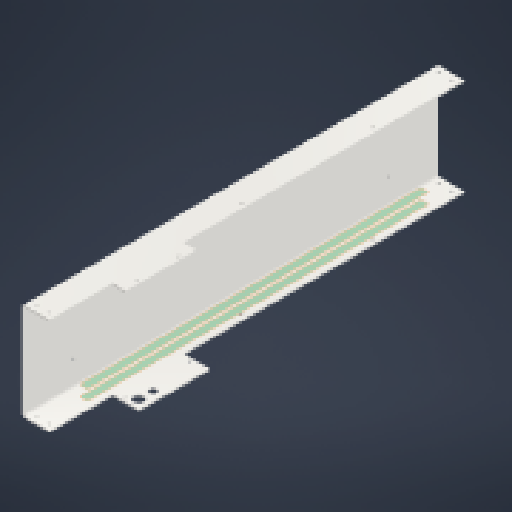
# Autodesk Inventor part: U-Blech-Bild
Saved by Autodesk Inventor 2026.1 (Build 301233020, 233B)
## iProperties
Created: 2025-04-28
Part Number: U-Blech-Bild
Material: Stahl, unlegiert
Document SubType Name: Sheet Metal
Designer: iopeter
Density: 7.85 g/cm^3
Sheet Metal Rule: Standard_mm
Appearance: Stahl
Author: iopeter
Autodesk Inventor part; units mm, degrees
ref_plane "YZ Plane" through (0, 0, 0) normal (1, 0, 0) x (0, 1, 0)
ref_plane "XZ Plane" through (0, 0, 0) normal (0, 1, 0) x (-1, 0, 0)
ref_plane "XY Plane" through (0, 0, 0) normal (0, 0, 1) x (1, 0, 0)
sketch "Skizze1" plane through (0, 0, 0) normal (0, 0, 1) x (1, 0, 0)
  line L0 (26.7, -375) -> (-26.6, -375)
  line L1 (-26.6, -375) -> (-26.6, 415)
  line L2 (-26.6, 415) -> (26.7, 415)
  line L3 (26.7, 415) -> (26.7, -375)
  line L4 (26.7, -120) -> (51.7, -120)
  line L5 (51.7, -120) -> (51.7, -255)
  line L6 (51.7, -255) -> (26.7, -255)
  line L7 (26.7, -255) -> (26.7, -120)
  line L8 (44.7, -147) -> (44.7, -148) construction
  line L9 (42.2, -147) -> (42.2, -148)
  line L10 (47.2, -148) -> (47.2, -147)
  arc A0 (47.2, -147) -> (42.2, -147) centre (44.7, -147) ccw
  arc A1 (42.2, -148) -> (47.2, -148) centre (44.7, -148) ccw
  line L11 (44.7, -227) -> (44.7, -228) construction
  line L12 (42.2, -227) -> (42.2, -228)
  line L13 (47.2, -228) -> (47.2, -227)
  arc A2 (47.2, -227) -> (42.2, -227) centre (44.7, -227) ccw
  arc A3 (42.2, -228) -> (47.2, -228) centre (44.7, -228) ccw
  line L14 (57.888, -187.5) -> (31.6499, -187.5) construction
  line L15 (16.7, 278.8638) -> (16.7, -278.8638) construction
  circle A4 centre (16.7, 250) radius 3
  circle A5 centre (16.7, 0) radius 3
  circle A6 centre (16.7, -250) radius 3
  point P0 (0, 0)
  point P1 (44.7, -147.5)
  point P2 (44.7, -227.5)
  dimension "d17" = 135
  dimension "d19" = 1
  dimension "d20" = 5
  dimension "d21" = 1
  dimension "d22" = 5
  dimension "d23" = 7
  dimension "d24" = 80
  dimension "d26" = 250
  dimension "d28" = 6
  dimension "d29" = 6
  dimension "d30" = 6
  dimension "d52" = 120
  dimension "d63" = 790
  dimension "d65" = 25
  dimension "d67" = 53.3
  dimension "d68" = 375
  dimension "d69" = 26.6
  dimension "d70" = 10
  dimension "d71" = 250
  measures "d17" distance between parallel lines of L6 L4
  measures "d19" distance of L8.start L8.end
  measures "d20" diameter of A1
  measures "d21" distance of L11.start L11.end
  measures "d22" diameter of A3
  measures "d23" distance from line of L5 point (44.7, -147.5)
  measures "d24" distance of point (44.7, -227.5) point (44.7, -147.5)
  measures "d26" distance of point (16.7, 250) point (16.7, 0)
  measures "d28" diameter of A4
  measures "d29" diameter of A5
  measures "d30" diameter of A6
  measures "d52" distance between parallel lines of L0 L6
  measures "d63" distance between parallel lines of L2 L0
  measures "d65" distance between parallel lines of L3 L5
  measures "d67" distance between parallel lines of L1 L3
  measures "d68" distance from line of point (0, 0) L0
  measures "d69" distance from line of L1 point (0, 0)
  measures "d70" distance between parallel lines of L3 L15
  measures "d71" vertical distance of point (0, 0) A6.centre
extrude "Grobblech1" add sketch "Skizze1" along normal blind 3 contours L0 L1 L2 L3 | L3 L4 L5 L6 | A6
ref_plane "Arbeitsebene1" through (13.4, 0, -160) normal (0, 0, -1) x (-1, 0, 0)
ref_plane "Work Plane2" through (13.4, 0, -180) normal (0, 0, -1) x (-1, 0, 0)
sketch "Skizze2" plane through (13.4, 0, -180) normal (0, 0, -1) x (-1, 0, 0)
  circle A0 centre (-3.3, 250) radius 3
  circle A1 centre (-3.3, 0) radius 3
  circle A2 centre (-3.3, -250) radius 3
  circle A3 centre (-3.3, 250) radius 3
  circle A4 centre (-3.3, 0) radius 3
  arc A5 (-33.8, -228) -> (-28.8, -228) centre (-31.3, -228) ccw construction
  line L0 (-28.8, -228) -> (-28.8, -227) construction
  arc A6 (-28.8, -227) -> (-33.8, -227) centre (-31.3, -227) ccw construction
  line L1 (-33.8, -227) -> (-33.8, -228) construction
  line L2 (-33.8, -147) -> (-33.8, -148) construction
  arc A7 (-33.8, -148) -> (-28.8, -148) centre (-31.3, -148) ccw construction
  line L3 (-28.8, -148) -> (-28.8, -147) construction
  arc A8 (-28.8, -147) -> (-33.8, -147) centre (-31.3, -147) ccw construction
  line L4 (-38.3, -120) -> (-38.3, -255)
  line L5 (-13.3, -120) -> (-38.3, -120)
  line L6 (-13.3, 415) -> (-13.3, -120)
  line L7 (40, 415) -> (-13.3, 415)
  line L8 (40, -375) -> (40, 415)
  line L9 (-13.3, -375) -> (40, -375)
  line L10 (-13.3, -255) -> (-13.3, -375)
  line L11 (-38.3, -255) -> (-13.3, -255)
  line L12 (-38.3, -255) -> (-63.3, -255)
  line L13 (-63.3, -255) -> (-63.3, -120)
  line L14 (-63.3, -120) -> (-38.3, -120)
  line L15 (-38.3, -120) -> (-38.3, -255)
  circle A9 centre (-45.3, -237) radius 10.375
  line L16 (-46.078, -226.6542) -> (-44.522, -226.6542)
  line L17 (-31.3, -228) -> (-31.3, -262.846) construction
  circle A10 centre (-31.3, -249) radius 2.5
  line L18 (-38.3, -255) -> (-38.3, -120)
  line L19 (-38.3, -187.5) -> (-17.972, -187.5) construction
  line L20 (-31.3, -147) -> (-31.3, -112.154) construction
  circle A11 centre (-31.3, -126) radius 2.5
  circle A12 centre (-45.3, -210) radius 8.05
  circle A13 centre (-45.3, -210) radius 11 construction
  line L21 (-55.8532, -247.1825) -> (-59.3949, -232.9519) construction
  line L22 (-59.3949, -232.9519) -> (-48.8417, -222.7694) construction
  line L23 (-48.8417, -222.7694) -> (-34.7468, -226.8175) construction
  line L24 (-34.7468, -226.8175) -> (-31.2051, -241.0481) construction
  line L25 (-31.2051, -241.0481) -> (-41.7583, -251.2306) construction
  line L26 (-41.7583, -251.2306) -> (-55.8532, -247.1825) construction
  circle A14 centre (-45.3, -237) radius 14.6647 construction
  line L27 (-37.25, -203.225) -> (-53.35, -203.225)
  line L28 (-53.35, -203.225) -> (-53.35, -216.775)
  line L29 (-53.35, -216.775) -> (-37.25, -216.775)
  line L30 (-37.25, -216.775) -> (-37.25, -203.225)
  line L31 (-37.25, -203.225) -> (-53.35, -216.775) construction
  line L32 (-53.35, -203.225) -> (-37.25, -216.775) construction
  line L33 (-50.7634, -228.18) -> (-39.8366, -228.18)
  point P0 (13.4, 0)
  point P1 (-38.3, -244.6577)
  point P2 (-38.3, -229.3423)
  point P3 (-53.35, -210)
  point P4 (-49.6476, -203.225)
  point P5 (-40.9524, -203.225)
  point P6 (-40.9524, -216.775)
  point P7 (-49.6476, -216.775)
  dimension "d53" = 25
  dimension "d55" = 20.75
  dimension "d57" = 18
  dimension "d58" = 18
  dimension "d59" = 5
  dimension "d60" = 6
  dimension "d61" = 16.1
  dimension "d62" = 27
  dimension "d75" = 22
  dimension "d76" = 25.4
  dimension "d77" = 13.55
  dimension "d78" = 8.82
  measures "d53" distance of L13.end L14.end
  measures "d55" diameter of A9
  measures "d57" distance from line of L13 A9.centre
  measures "d58" distance from line of L12 A9.centre
  measures "d59" diameter of A10
  measures "d60" distance from line of L11 A10.centre
  measures "d61" diameter of A12
  measures "d62" distance of A9.centre A12.centre
  measures "d75" diameter of A13
  measures "d76" distance between parallel lines of L24 L21
  measures "d77" distance between parallel lines of L27 L29
  measures "d78" distance from line of A9.centre L33
sheet face with bend "Fläche2" sketch "Skizze2" thickness 3 toward (0, 0, -1) bend radius 3 contours A2 | L5 L6 L7 L8 L9 L10 L11 L4 A9 L29 L30 L27 | L4 L27 A12 L28 L29 A9 L12 L13 L14 | L27 L30 A12 L4 | L4 A12 L27 | A12 L4 | L27 A12 | A12 L30 L29 L4 | L4 L29 A12 | A12 L28 L27 | A12 L29 | A12 L29 L28 | A9 L16 L33
bend "Biegung1"
sketch "Skizze4" plane through (-26.6, -375, -180) normal (-1, 0, 0) x (0, 0, 1)
  line L0 (0, 0) -> (0, 790)
  line L1 (180, 790) -> (180, 0)
  line L2 (0, 790) -> (180, 790)
  line L3 (0, 120) -> (0, 0)
  line L4 (0, 0) -> (180, 0)
  point P0 (180, 375)
sheet face with bend "Fläche4" sketch "Skizze4" thickness 3 toward (1, 0, 0) bend radius 3
bend "Biegung3"
sketch "Skizze5" plane through (0, 0, 3) normal (0, 0, 1) x (1, 0, 0)
  line L0 (20.2658, 403) -> (-16.6894, 403) construction
  line L1 (-26.6, 415) -> (26.7, 415) projected
  circle A0 centre (14.7, 403) radius 3
  circle A1 centre (-10.3, 403) radius 3
  line L2 (0, 480.3332) -> (0, 464.4547) construction
  point P0 (0, 0)
  point P1 (-20.6, 415)
  dimension "d36" = 12
  dimension "d37" = 6
  dimension "d38" = 6
  dimension "d39" = 25
  constraints: 4 end point, 2 centre point, 2 point on line, 1 horizontal, 1 vertical, 1 vertical alignment
  measures "d36" distance between parallel lines of L1 L0
  measures "d37" diameter of A0
  measures "d38" diameter of A1
  measures "d39" distance of A1.centre A0.centre
extrude "Extrusion1" cut sketch "Skizze5" against normal through all
sketch "Skizze6" plane through (-26.6, -375, -180) normal (-1, 0, 0) x (0, 0, 1)
  line L0 (177, 790) -> (3, 790) projected
  line L1 (90, 790) -> (90, 0) construction
  line L2 (3, 0) -> (177, 0) projected
  line L3 (177, 0) -> (177, 790) projected
  line L4 (177, 395) -> (3, 395) construction
  line L5 (3, 790) -> (3, 0) projected
  line L6 (45, 95) -> (135, 95) construction
  line L7 (135, 95) -> (135, 695) construction
  line L8 (135, 695) -> (45, 695) construction
  line L9 (45, 695) -> (45, 95) construction
  line L10 (45, 95) -> (135, 695) construction
  line L11 (135, 95) -> (45, 695) construction
  circle A0 centre (135, 695) radius 3
  circle A1 centre (135, 95) radius 3
  circle A2 centre (45, 95) radius 3
  circle A3 centre (45, 695) radius 3
  point P0 (180, 375)
  point P1 (90, 395)
  dimension "d43" = 90
  dimension "d44" = 600
  dimension "d45" = 6
  dimension "d46" = 6
  dimension "d47" = 6
  dimension "d48" = 6
  constraints: 16 end point, 7 midpoint, 4 centre point, 4 coincident, 2 parallel, 1 horizontal, 1 perpendicular
  measures "d43" distance of L8.end L7.end
  measures "d44" distance of L7.end L6.end
  measures "d45" diameter of A0
  measures "d46" diameter of A1
  measures "d47" diameter of A2
  measures "d48" diameter of A3
extrude "Extrusion2" cut sketch "Skizze6" against normal through all contours A0 | A1 | A2 | A3
move or copy body "Körper verschieben1" bodies to move or copy 1 copy no translate (0, -35, 0)
sketch "Sketch7" plane through (76.7, -155, -183) normal (0, 0, -1) x (-1, 0, 0)
  line L0 (53.3099, -243) -> (92.7727, -243) construction
  line L1 (97.3, -255) -> (50, -255) construction
  circle A0 centre (62, -243) radius 2.5
  circle A1 centre (87, -243) radius 2.5
  line L2 (50, -255) -> (50, -135) construction
  point P0 (76.7, 155)
  dimension "d79" = 12
  dimension "d80" = 5
  dimension "d81" = 5
  dimension "d82" = 12
  dimension "d83" = 25
  constraints: 2 centre point, 2 end point, 2 point on line, 1 horizontal
  measures "d79" distance between parallel lines of L1 L0
  measures "d80" diameter of A0
  measures "d81" diameter of A1
  measures "d82" distance from line of L2 A0.centre
  measures "d83" distance of A1.centre A0.centre
extrude "Extrusion3" cut sketch "Sketch7" against normal through all
equation "\"d2\" = Stärke"
equation "\"d6\" = Biegeradius"
equation "\"d7\" = BreiteBiegungsfreistellung"
equation "\"d9\" = MinimalRest"
equation "\"d8\" = TiefeBiegungsfreistellung"
equation "\"d10\" = Übergangsradius"
equation "\"d31\" = Biegeradius"
equation "\"d32\" = BreiteBiegungsfreistellung"
equation "\"d34\" = MinimalRest"
equation "\"d33\" = TiefeBiegungsfreistellung"
equation "\"d35\" = Übergangsradius"
equation "\"Biegeradius\" = Stärke"
equation "\"BreiteBiegungsfreistellung\" = Stärke"
equation "\"TiefeBiegungsfreistellung\" = 0.5 * Stärke"
equation "\"GrößeEckenfreistellung\" = 4 * Stärke"
equation "\"MinimalRest\" = 2 * Stärke"
equation "\"Übergangsradius\" = Biegeradius"
equation "\"JacobiRadiusGröße\" = Biegeradius"
equation "\"Abstandsgröße\" = Stärke"
equation "\"Stärke\" = 3"
